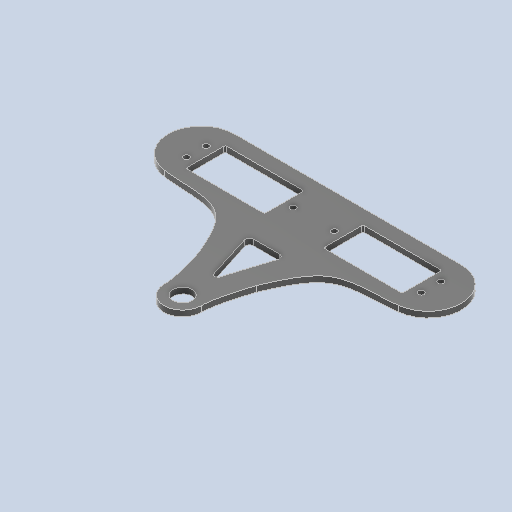
# Autodesk Inventor part: Shoulder_bottom
Saved by Autodesk Inventor 2023.1 (Build 271208000, 208)
## iProperties
Created: 2022-08-10
Part Number: Shoulder_bottom
Material: Thermoplastic Resin
Document SubType Name: Modeling
Designer: Windows10
Density: 1.28 g/cm^3
Appearance: Smooth - Black
Author: Windows10
Autodesk Inventor part; units mm, degrees
ref_plane "YZ Plane" through (0, 0, 0) normal (1, 0, 0) x (0, 1, 0)
ref_plane "XZ Plane" through (0, 0, 0) normal (0, 1, 0) x (-1, 0, 0)
ref_plane "Work Plane7" through (3.7071, 39.9, 0.5) normal (0, 1, 0) x (1, 0, 0)
sketch "Sketch4" plane through (3.7071, 39.9, 0.5) normal (0, 1, 0) x (1, 0, 0)
  circle A0 centre (6.2928, -9.3) radius 2.9
  circle A1 centre (6.2928, -9.3) radius 2.65
  line L0 (6.2928, -9.3) -> (6.2928, -8.1563)
  circle A2 centre (6.2928, -9.3) radius 1.5
  line L1 (5.9607, -6.6709) -> (6.3303, -6.4003)
  line L2 (6.6249, -6.6709) -> (6.3303, -6.4003)
  line L3 (5.3173, -6.8361) -> (5.608, -6.482)
  line L4 (5.9607, -6.6709) -> (5.608, -6.482)
  line L5 (4.7352, -7.1561) -> (4.9287, -6.7409)
  line L6 (5.3173, -6.8361) -> (4.9287, -6.7409)
  line L7 (4.2509, -7.6109) -> (4.3351, -7.1605)
  line L8 (4.7352, -7.1561) -> (4.3351, -7.1605)
  line L9 (3.895, -8.1717) -> (3.8646, -7.7146)
  line L10 (4.2509, -7.6109) -> (3.8646, -7.7146)
  line L11 (3.6897, -8.8035) -> (3.5466, -8.3682)
  line L12 (3.895, -8.1717) -> (3.5466, -8.3682)
  line L13 (3.648, -9.4664) -> (3.4011, -9.0805)
  line L14 (3.6897, -8.8035) -> (3.4011, -9.0805)
  line L15 (3.7725, -10.1189) -> (3.4374, -9.8065)
  line L16 (3.648, -9.4664) -> (3.4374, -9.8065)
  line L17 (4.0553, -10.72) -> (3.653, -10.5007)
  line L18 (3.7725, -10.1189) -> (3.653, -10.5007)
  line L19 (4.4787, -11.2318) -> (4.0346, -11.1195)
  line L20 (4.0553, -10.72) -> (4.0346, -11.1195)
  line L21 (5.0161, -11.6222) -> (4.558, -11.6239)
  line L22 (4.4787, -11.2318) -> (4.558, -11.6239)
  line L23 (5.6338, -11.8668) -> (5.1904, -11.9823)
  line L24 (5.0161, -11.6222) -> (5.1904, -11.9823)
  line L25 (6.2928, -11.95) -> (5.8921, -12.1722)
  line L26 (5.6338, -11.8668) -> (5.8921, -12.1722)
  line L27 (6.9518, -11.8668) -> (6.619, -12.1816)
  line L28 (6.2928, -11.95) -> (6.619, -12.1816)
  line L29 (7.5694, -11.6222) -> (7.3254, -12.01)
  line L30 (6.9518, -11.8668) -> (7.3254, -12.01)
  line L31 (8.1068, -11.2318) -> (7.9668, -11.6681)
  line L32 (7.5694, -11.6222) -> (7.9668, -11.6681)
  line L33 (8.5303, -10.72) -> (8.5032, -11.1773)
  line L34 (8.1068, -11.2318) -> (8.5032, -11.1773)
  line L35 (8.8131, -10.1189) -> (8.9006, -10.5687)
  line L36 (8.5303, -10.72) -> (8.9006, -10.5687)
  line L37 (8.9376, -9.4664) -> (9.1341, -9.8803)
  line L38 (8.8131, -10.1189) -> (9.1341, -9.8803)
  line L39 (8.8959, -8.8035) -> (9.1892, -9.1554)
  line L40 (8.9376, -9.4664) -> (9.1892, -9.1554)
  line L41 (8.6906, -8.1717) -> (9.0622, -8.4397)
  line L42 (8.8959, -8.8035) -> (9.0622, -8.4397)
  line L43 (8.3346, -7.6109) -> (8.7613, -7.778)
  line L44 (8.6906, -8.1717) -> (8.7613, -7.778)
  line L45 (7.8504, -7.1561) -> (8.3052, -7.2119)
  line L46 (8.3346, -7.6109) -> (8.3052, -7.2119)
  line L47 (7.2683, -6.8361) -> (7.7227, -6.777)
  line L48 (7.8504, -7.1561) -> (7.7227, -6.777)
  line L49 (6.6249, -6.6709) -> (7.0503, -6.5007)
  line L50 (7.2683, -6.8361) -> (7.0503, -6.5007)
  line L51 (-48.7072, 67.5) -> (-9.1072, 67.5)
  line L52 (-9.1072, 67.5) -> (-9.1072, 47.9)
  line L53 (-9.1072, 47.9) -> (-48.7072, 47.9)
  line L54 (-48.7072, 47.9) -> (-48.7072, 67.5)
  line L55 (-9.6072, 67.8) -> (-48.2072, 67.8)
  line L56 (-49.0072, 67) -> (-49.0072, 48.4)
  line L57 (-48.2072, 47.6) -> (-9.6072, 47.6)
  line L58 (-8.8072, 48.4) -> (-8.8072, 67)
  arc A3 (-48.2072, 67.8) -> (-49.0072, 67) centre (-48.2072, 67) ccw
  arc A4 (-49.0072, 48.4) -> (-48.2072, 47.6) centre (-48.2072, 48.4) ccw
  arc A5 (-8.8072, 67) -> (-9.6072, 67.8) centre (-9.6072, 67) ccw
  arc A6 (-9.6072, 47.6) -> (-8.8072, 48.4) centre (-9.6072, 48.4) ccw
  circle A7 centre (-38.7072, 57.7) radius 2.8043
  line L59 (-28.9072, 67.5) -> (-28.9072, 60.5718)
  arc A8 (-51.4012, 75.2248) -> (-53.5593, 41.3351) centre (-51.641, 58.2265) ccw
  arc A9 (14.1928, -9.3) -> (-1.6072, -9.3) centre (6.2928, -9.3) ccw
  line L60 (-53.5593, 41.3351) -> (-46.7288, 40.1839) construction
  line L61 (-46.7288, 40.1839) -> (-26.4146, 41.3143) construction
  line L62 (-26.4146, 41.3143) -> (-16.8338, 33.5272) construction
  line L63 (-16.8338, 33.5272) -> (-7.2254, 12.1154) construction
  line L64 (-7.2254, 12.1154) -> (-2.9491, -1.4) construction
  line L65 (-2.9491, -1.4) -> (-1.6072, -5.4747) construction
  line L66 (-1.6072, -5.4747) -> (-1.6072, -9.3) construction
  spline S0 degree 4 poles (-53.5593, 41.3351) (-46.7288, 40.1839) (-26.4146, 41.3143) (-16.8338, 33.5272) (-7.2254, 12.1154) (-2.9491, -1.4) (-1.6072, -5.4747) (-1.6072, -9.3) knots 1 1 1 1 1 2 3 4 5 5 5 5 5
  line L67 (61.2928, 67.5) -> (21.6928, 67.5)
  line L68 (21.6928, 67.5) -> (21.6928, 47.9)
  line L69 (21.6928, 47.9) -> (61.2928, 47.9)
  line L70 (61.2928, 47.9) -> (61.2928, 67.5)
  line L71 (22.1928, 67.8) -> (60.7928, 67.8)
  line L72 (61.5928, 67) -> (61.5928, 48.4)
  line L73 (60.7928, 47.6) -> (22.1928, 47.6)
  line L74 (21.3928, 48.4) -> (21.3928, 67)
  arc A10 (61.5928, 67) -> (60.7928, 67.8) centre (60.7928, 67) ccw
  arc A11 (60.7928, 47.6) -> (61.5928, 48.4) centre (60.7928, 48.4) ccw
  arc A12 (22.1928, 67.8) -> (21.3928, 67) centre (22.1928, 67) ccw
  arc A13 (21.3928, 48.4) -> (22.1928, 47.6) centre (22.1928, 48.4) ccw
  circle A14 centre (51.2928, 57.7) radius 2.8043
  line L75 (41.4928, 67.5) -> (41.4928, 60.5718)
  arc A15 (66.1449, 41.3351) -> (63.9868, 75.2248) centre (64.2266, 58.2265) ccw
  line L76 (66.1449, 41.3351) -> (59.3144, 40.1839) construction
  line L77 (59.3144, 40.1839) -> (39.0002, 41.3143) construction
  line L78 (39.0002, 41.3143) -> (29.4194, 33.5272) construction
  line L79 (29.4194, 33.5272) -> (19.811, 12.1154) construction
  line L80 (19.811, 12.1154) -> (15.5347, -1.4) construction
  line L81 (15.5347, -1.4) -> (14.1928, -5.4747) construction
  line L82 (14.1928, -5.4747) -> (14.1928, -9.3) construction
  spline S1 degree 4 poles (66.1449, 41.3351) (59.3144, 40.1839) (39.0002, 41.3143) (29.4194, 33.5272) (19.811, 12.1154) (15.5347, -1.4) (14.1928, -5.4747) (14.1928, -9.3) knots 1 1 1 1 1 2 3 4 5 5 5 5 5
  arc A16 (-1.6072, -9.3) -> (14.1928, -9.3) centre (6.2928, -9.3) ccw
  circle A17 centre (-53.6572, 62.7) radius 1.5
  line L83 (-49.0072, 57.7) -> (-54.6618, 57.7)
  circle A18 centre (-53.6572, 52.7) radius 1.5
  circle A19 centre (66.2428, 62.7) radius 1.5
  circle A20 centre (66.2428, 52.7) radius 1.5
  circle A21 centre (6.2928, -9.3) radius 4.95
  line L84 (-4.1572, 57.7) -> (-3.4323, 57.7)
  circle A22 centre (-4.1572, 57.7) radius 1.5
  circle A23 centre (16.7428, 57.7) radius 1.5
  line L85 (-51.4012, 75.2248) -> (63.9868, 75.2248)
  circle A24 centre (6.2928, -9.3) radius 9.5
  line L86 (-3.2072, -9.3) -> (-3.2072, -6.2163) construction
  line L87 (-3.2072, -6.2163) -> (-3.7947, -2.1829) construction
  line L88 (-3.7947, -2.1829) -> (-5.6572, 5.3052) construction
  line L89 (-5.6572, 5.3052) -> (-8.4358, 13.8026) construction
  spline S2 degree 4 poles (-3.2072, -9.3) (-3.2072, -6.2163) (-3.7947, -2.1829) (-5.6572, 5.3052) (-8.4358, 13.8026) knots 1 1 1 1 1 2 2 2 2 2
  line L90 (15.7928, -9.3) -> (15.7928, -6.2163) construction
  line L91 (15.7928, -6.2163) -> (16.3803, -2.1829) construction
  line L92 (16.3803, -2.1829) -> (18.2428, 5.3052) construction
  line L93 (18.2428, 5.3052) -> (21.0213, 13.8026) construction
  spline S3 degree 4 poles (15.7928, -9.3) (15.7928, -6.2163) (16.3803, -2.1829) (18.2428, 5.3052) (21.0213, 13.8026) knots 1 1 1 1 1 2 2 2 2 2
  line L94 (6.2928, 52.7) -> (6.2928, 2.4423)
  line L95 (6.2928, 33.5913) -> (-0.4039, 33.5913)
  line L96 (-2.3125, 30.9937) -> (6.2928, 3.511)
  arc A25 (-0.4039, 33.5913) -> (-2.3125, 30.9937) centre (-0.4039, 31.5913) ccw
  line L97 (6.2928, 33.5913) -> (12.9895, 33.5913)
  line L98 (14.8981, 30.9937) -> (6.2928, 3.511)
  arc A26 (14.8981, 30.9937) -> (12.9895, 33.5913) centre (12.9895, 31.5913) ccw
  arc A27 (4.7409, 8.4673) -> (7.8447, 8.4673) centre (6.2928, 8.7018) ccw
  point P0 (6.2928, -6.65)
  point P1 (-28.9072, 64.0359)
  point P2 (41.4928, 64.0359)
  point P3 (8.8959, -8.8035)
  point P4 (8.8131, -10.1189)
  point P5 (8.1068, -11.2318)
  point P6 (7.5694, -11.6222)
  point P7 (6.6249, -6.6709)
  point P8 (8.9006, -10.5687)
  point P9 (3.4374, -9.8065)
  point P10 (8.9006, -10.5687)
  point P11 (3.4374, -9.8065)
  point P12 (3.653, -10.5007)
  point P13 (7.9668, -11.6681)
  point P14 (3.653, -10.5007)
  point P15 (7.3254, -12.01)
  point P16 (7.9668, -11.6681)
  point P17 (6.619, -12.1816)
  point P18 (7.3254, -12.01)
  point P19 (6.619, -12.1816)
  point P20 (6.2928, -17.2)
  point P21 (21.0213, 13.8026)
  point P22 (7.7013, 8.0093)
  point P23 (4.8843, 8.0093)
  dimension "d26" = 5.8
  dimension "d105" = 19
  dimension "d31" = 0.25
  dimension "d32" = 3
  dimension "d36" = 360
  dimension "d68" = 45
  dimension "d69" = 67
  dimension "d70" = 39.6
  dimension "d71" = 19.6
  dimension "d72" = 10
  dimension "d73" = 9.8
  dimension "d74" = 0.3
  dimension "d75" = 0.8
  dimension "d78" = 5
  dimension "d91" = 24.75
  dimension "d92" = 3
  dimension "d93" = 5
  dimension "d99" = 9.9
  dimension "d102" = 3
  dimension "d104" = 17
  dimension "d106" = 2
  constraints: 154 end point, 34 point on circle, 26 centre point, 11 tangent, 8 coincident, 5 horizontal, 5 symmetric about line, 5 vertical, 4 parallel, 4 point on line, 3 equal radius, 3 midpoint, 2 perpendicular, 150 other
  measures "d32" diameter of A2
  measures "d68" horizontal distance of point (-38.707, 57.7) A2.centre
  measures "d69" vertical distance of L0.start point (-38.707, 57.7)
  measures "d70" distance of L51.start L51.end
  measures "d71" distance of L51.end L52.end
  measures "d72" distance from line of L54 point (-38.707, 57.7)
  measures "d73" distance from line of L51 point (-38.707, 57.7)
  measures "d74" distance between parallel lines of L51 L55
  measures "d75" radius of A3
  measures "d91" distance from line of L59 A17.centre
  measures "d92" diameter of A17
  measures "d93" distance from line of L83 A17.centre
  measures "d99" diameter of A21
  measures "d102" diameter of A22
  measures "d104" radius of A8
  measures "d106" radius of A25
extrude "Extrusion9" add sketch "Sketch4" along normal blind 3 contours L85 A15 S1 A24 S0 A8 | S0 A24 S2 | A24 S1 A9 S0 | S0 A16 S1 A24 | S3 A24 S1 | A9 A16 | A27 L98 L94 | L94 L96 A27 | A27 L96 | L98 A27
equation "\"d73\" = 0.5 * d71"
body "Solid4"
